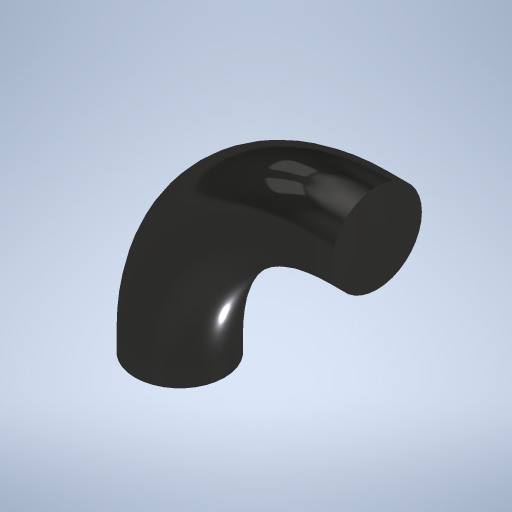
# Autodesk Inventor part: cable 90°
Saved by Autodesk Inventor 2023 (Build 270158000, 158)
## iProperties
Created: 2022-10-27
Part Number: cable 90°
Material: Generic
Document SubType Name: Modeling
Designer: Xiaba
Density: 1 g/cm^3
Appearance: Default
Author: Xiaba
Autodesk Inventor part; units mm, degrees
ref_plane "YZ Plane" through (0, 0, 0) normal (1, 0, 0) x (0, 1, 0)
ref_plane "XZ Plane" through (0, 0, 0) normal (0, 1, 0) x (-1, 0, 0)
ref_plane "XY Plane" through (0, 0, 0) normal (0, 0, 1) x (1, 0, 0)
sketch "Sketch1" plane through (0, 0, 0) normal (0, 1, 0) x (-1, 0, 0)
  circle A0 centre (0, 0) radius 0.25
  dimension "d0" = 0.5
  constraints: 1 centre point, 1 coincident
  measures "d0" diameter of A0
sketch "Sketch2" plane through (0, 0, 0) normal (0, 0, 1) x (1, 0, 0)
  line L0 (0, 0) -> (0, 0)
  line L1 (1, 1) -> (1, 1)
  arc A0 (1, 1) -> (0, 0) centre (1, 0) ccw
  point P0 (0, 1)
  dimension "d1" = 1
  dimension "d2" = 1
  dimension "d3" = 1
  constraints: 4 end point, 2 point on circle, 2 point on line, 2 tangent, 1 centre point, 1 perpendicular, 1 vertical
  measures "d1" distance of L0.start point (0, 1)
  measures "d2" distance of point (0, 1) L1.end
  measures "d3" radius of A0
sweep "Sweep1" add profiles "Sketch1" path "Sketch2" path curves A0
sketch "Sketch3" plane through (1, 1, 0) normal (1, 0, 0) x (0, 0, -1)
  circle A0 centre (0, 0) radius 0.25 projected
  point P0 (0, -1)
extrude "Extrusion1" add sketch "Sketch3" along normal blind 0.1
sketch "Sketch4" plane through (0, 0, 0) normal (0, -1, 0) x (1, 0, 0)
  circle A0 centre (0, 0) radius 0.25 projected
extrude "Extrusion2" add sketch "Sketch4" along normal blind 0.1
body "Solid1"
